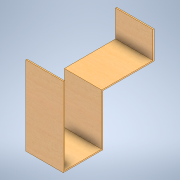
# Autodesk Inventor part: Body Skeleton
Saved by Autodesk Inventor 2022.2 (Build 262287000, 287)
## iProperties
Created: 2022-02-23
Part Number: Body Skeleton
Material: Pine, Southern
Document SubType Name: Modeling
Designer: PRASHANTH
Density: 0.570257 g/cm^3
Appearance: Yellow Pine - Stained Dark Medium Gloss
Author: PRASHANTH
Autodesk Inventor part; units mm, degrees
ref_plane "YZ Plane" through (0, 0, 0) normal (1, 0, 0) x (0, 1, 0)
ref_plane "XZ Plane" through (0, 0, 0) normal (0, 1, 0) x (-1, 0, 0)
ref_plane "XY Plane" through (0, 0, 0) normal (0, 0, 1) x (1, 0, 0)
sketch "Sketch1" plane through (0, 0, 0) normal (1, 0, 0) x (0, 1, 0)
  line L0 (-50, 110) -> (-50, -110)
  line L1 (-50, -110) -> (45, -110)
  line L2 (-50, 110) -> (-270, 110)
  line L3 (-270, 110) -> (-270, 280)
  line L4 (-270, 280) -> (70, 280)
  line L5 (70, -105) -> (-45, -105)
  line L6 (-45, -105) -> (-45, 115)
  line L7 (-45, 115) -> (-265, 115)
  line L8 (-265, 115) -> (-265, 275)
  line L9 (-265, 275) -> (45, 275)
  line L10 (-50, -110) -> (70, -110)
  line L11 (70, -110) -> (70, -105)
  line L12 (70, 275) -> (70, 280)
  line L13 (45, 275) -> (70, 275)
  point P0 (0, 0)
  constraints: 28 end point, 3 perpendicular, 3 vertical, 1 horizontal, 1 point on line, 2 other
extrude "Extrusion1" add sketch "Sketch1" along normal blind 160
body "Solid1"
